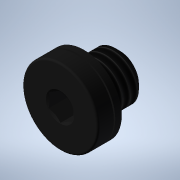
# Autodesk Inventor part: 174308 B-M5-B
Saved by Autodesk Inventor 2021 (Build 250183000, 183)
## iProperties
Created: 2026-04-25
Part Number: 174308 B-M5-B
Material: Generic
Catalog Web Link: www.3dfindit.com
Description: B-blanking plug
Vendor: FESTO
Document SubType Name: Modeling
Designer: psAdmin
Manufacturer: FESTO
Mass: 1 g
Surface Area: 2.64835 cm^2
Volume: 0.181472 cm^3
Density: 1 g/cm^3
Appearance: PSOLRGB-128-128-128
Category: PARTsolutions
Company: FESTO
Title: 174308 B-M5-B
Author: Cadenas PARTsolutions
Comments: blanking plug
PSOL_IDENT_0: {$CADENAS_DATA/23d-libs/festo/parts/b/b/b.prj},161 {VTYP=3D},{NB=174308 B-M5-B},{LINA=174308 B-M5-B}
PSOL_IDENT_1: ,{NN=B},{DATE=30.04.2025 13:57:12},{GEOMDATE=18.03.2025 13:12:43},{VERSION=},{LINEID=40},{WBVAR=},{W
PSOL_IDENT_2: BNUMERIC=}  {NB=174308 B-M5-B},{LINA=174308 B-M5-B},{KT=DUMMY},{TNR=174308},{TYP=B-M5-B},{VERS=3.000
PSOL_IDENT_3: },{BR=0.000},{L=6.300},{L1=2.500},{B=3.800},{A=8.000},{D=M5},{SW1=0.000},{SW2=2.500},{DNDR=5.000},{D
PSOL_IDENT_4: M=1},{CNSMASSEXACT=0.001},{GTIN=4052568004811},{REACH=Ja},{REACHSVHC=Ja},{REACHHAZSUBS=7439-92-1},{R
PSOL_IDENT_5: EACHSCIP=d30196e2-cd10-461a-bddb-17e770d92110,1489ff2d-9e72-48bb-84ed-acc4fab91a2c},{REACHVALDATE=05
PSOL_IDENT_6: .03.2025}
NB: 174308 B-M5-B
NN: B
NT: blanking plug
NBSYN: $TNR. $TYP.
LINA: 174308 B-M5-B
CATALOG: Festo
TNR: 174308
TYP: B-M5-B
L: 6.3
L1: 2.5
B: 3.8
A: 8
D: M5
SW1: 0
SW2: 2.5
CNSMASSEXACT: 0.001
GTIN: 4052568004811
REACH: Yes
REACHSVHC: Yes
REACHHAZSUBS: 7439-92-1
REACHSCIP: d30196e2-cd10-461a-bddb-17e770d92110,1489ff2d-9e72-48bb-84ed-acc4fab91a2c
REACHVALDATE: 05.03.2025
SUPPLIER: FESTO
ARTICLENO: 174308 B-M5-B
BOMINFO: 174308 B-M5-B
CREATOR: CADENAS GmbH
Autodesk Inventor part; units mm, degrees
sketch "Sketch_1" plane through (0, 0, 0) normal (1, 0, 0) x (0, 1, 0)
  line L0 (0, -3.8) -> (0, 1.634)
  line L1 (0, 1.634) -> (1.5, 2.5)
  line L2 (1.5, 2.5) -> (3.8, 2.5)
  arc A0 (4, 2.3) -> (3.8, 2.5) centre (3.8, 2.3) ccw
  line L3 (4, 2.3) -> (4, 0.8333)
  line L4 (4, 0.8333) -> (3.6, 0.8333)
  line L5 (3.6, 0.8333) -> (3.6, 0.6833)
  line L6 (3.6, 0.6833) -> (4, 0.6833)
  line L7 (4, 0.6833) -> (4, 0)
  line L8 (4, 0) -> (2.0095, 0)
  line L9 (2.0095, 0) -> (2.5, -0.4905)
  line L10 (2.5, -0.4905) -> (2.5, -3.3095)
  line L11 (2.5, -3.3095) -> (2.0095, -3.8)
  line L12 (2.0095, -3.8) -> (0, -3.8)
  line L13 (0, -3.8) -> (0, 1.634)
  constraints: 28 end point, 2 point on circle, 1 centre point
revolve "Revolution1" add sketch "Sketch_1" angle 360 about axis through (0, 0, -3.8) along (0, 0, -1)
thread "Thread1" size "M5x0.8" class "6g" standard "ISO Metric profile" full length
sketch "Skizze_4" plane through (0, 0, 2.5) normal (0, 0, 1) x (1, 0, 0)
  line L0 (-1.25, -0.7217) -> (0, -1.4434)
  line L1 (0, -1.4434) -> (1.25, -0.7217)
  line L2 (1.25, -0.7217) -> (1.25, 0.7217)
  line L3 (1.25, 0.7217) -> (0, 1.4434)
  line L4 (0, 1.4434) -> (-1.25, 0.7217)
  line L5 (-1.25, 0.7217) -> (-1.25, -0.7217)
  constraints: 12 end point
extrude "Extrusion1" cut sketch "Skizze_4" against normal blind 2.5
ref_plane "ANBAU_XY" through (0, 0, 0) normal (0, 0, 1) x (1, 0, 0)
ref_plane "ANBAU_YZ" through (0, 0, 0) normal (1, 0, 0) x (0, 1, 0)
ref_plane "ANBAU_ZX" through (0, 0, 0) normal (0, 1, 0) x (0, 0, 1)
ref_plane "ANBAU_STD_XY" through (0, 0, 0) normal (0, 0, 1) x (1, 0, 0)
ref_plane "ANBAU_STD_YZ" through (0, 0, 0) normal (1, 0, 0) x (0, 1, 0)
ref_plane "ANBAU_STD_ZX" through (0, 0, 0) normal (0, 1, 0) x (0, 0, 1)
ref_plane "CPV_XY" through (0, 0, 0) normal (0, 0, 1) x (1, 0, 0)
ref_plane "CPV_YZ" through (0, 0, 0) normal (1, 0, 0) x (0, 1, 0)
ref_plane "CPV_ZX" through (0, 0, 0) normal (0, 1, 0) x (0, 0, 1)
body "Solid1"
